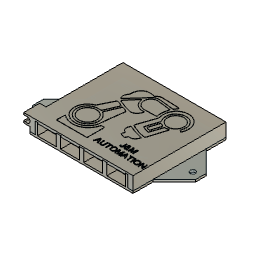
Box for ubs extension cable (Autodesk Fusion 360 design; units mm, degrees)
Autodesk Fusion 360 part; units mm, degrees
(part 1 of 2)
sketch "Sketch1" plane through (0, 0, 0) normal (0, 0, 1) x (1, 0, 0)
  line L0 (0, 0) -> (17, 0)
  line L1 (17, 0) -> (17, 9)
  line L2 (17, 9) -> (0, 9)
  line L3 (0, 9) -> (0, 0)
  line L4 (-0.35, -0.35) -> (17.35, -0.35)
  line L5 (17.35, -0.35) -> (17.35, 9.35)
  line L6 (17.35, 9.35) -> (-0.35, 9.35)
  line L7 (-0.35, 9.35) -> (-0.35, -0.35)
  line L8 (-0.35, 9.35) -> (17.35, 9.35)
  line L9 (17.35, 9.35) -> (17.35, 9.85)
  line L10 (17.35, 9.85) -> (-0.35, 9.85)
  line L11 (-0.35, 9.85) -> (-0.35, 9.35)
  line L12 (-0.35, 9.85) -> (0.65, 9.85)
  line L13 (0.65, 9.85) -> (0.65, 9.35)
  line L14 (0.65, 9.35) -> (-0.35, 9.35)
  line L15 (-0.35, 9.35) -> (-0.35, 9.85)
  line L16 (17.35, 9.85) -> (16.35, 9.85)
  line L17 (16.35, 9.85) -> (16.35, 9.35)
  line L18 (16.35, 9.35) -> (17.35, 9.35)
  line L19 (17.35, 9.35) -> (17.35, 9.85)
  line L20 (17.35, -0.35) -> (19.35, -0.35)
  line L21 (19.35, -0.35) -> (19.35, 9.85)
  line L22 (19.35, 9.85) -> (17.35, 9.85)
  line L23 (17.35, 9.85) -> (17.35, -0.35)
  line L24 (-0.35, -0.35) -> (-2.35, -0.35)
  line L25 (-2.35, -0.35) -> (-2.35, 9.85)
  line L26 (-2.35, 9.85) -> (-0.35, 9.85)
  line L27 (-0.35, 9.85) -> (-0.35, -0.35)
  line L28 (0.65, 9.85) -> (0.65, 9.35)
  line L29 (0.65, 9.35) -> (-0.35, 9.35)
  line L30 (-2.35, -0.35) -> (-2.35, 9.85)
  line L31 (-0.35, 9.85) -> (-0.35, -0.35)
  line L32 (0, 0) -> (17, 0)
  line L33 (17.35, 9.35) -> (17.35, 9.85)
  line L34 (19.35, -0.35) -> (19.35, 9.85)
  line L35 (17.35, -0.35) -> (17.35, 9.35)
  line L36 (17, 0) -> (17, 9)
  line L37 (17, 9) -> (0, 9)
  line L38 (0, 9) -> (0, 0)
  line L39 (-0.35, 9.35) -> (-0.35, -0.35)
  line L40 (17.35, 9.85) -> (-0.35, 9.85)
  line L41 (-0.35, 9.85) -> (-0.35, 9.35)
  line L42 (17.35, 9.85) -> (17.35, -0.35)
  line L43 (-0.35, -0.35) -> (-2.35, -0.35)
  line L44 (17.35, 9.35) -> (-0.35, 9.35)
  line L45 (17.35, 9.85) -> (16.35, 9.85)
  line L46 (-0.35, 9.35) -> (-0.35, 9.85)
  line L47 (17.35, -0.35) -> (19.35, -0.35)
  line L48 (16.35, 9.85) -> (16.35, 9.35)
  line L49 (-0.35, 9.85) -> (0.65, 9.85)
  line L50 (19.35, 9.85) -> (17.35, 9.85)
  line L51 (-2.35, 9.85) -> (-0.35, 9.85)
  line L52 (-0.35, 9.35) -> (17.35, 9.35)
  line L53 (-0.35, -0.35) -> (17.35, -0.35)
  line L54 (17.35, 9.35) -> (17.35, 9.85)
  line L55 (16.35, 9.35) -> (17.35, 9.35)
  line L56 (21.3167, 9.35) -> (21.3167, 9.85)
  line L57 (21.3167, 9.85) -> (22.3167, 9.85)
  line L58 (22.3167, 9.85) -> (22.3167, 9.35)
  line L59 (21.6667, 9) -> (21.6667, 0)
  line L60 (21.6667, 9) -> (21.6667, 0)
  line L61 (21.3167, 9.85) -> (21.3167, 9.35)
  line L62 (19.3167, -0.35) -> (19.3167, 9.85)
  line L63 (21.3167, -0.35) -> (19.3167, -0.35)
  line L64 (19.3167, 9.85) -> (21.3167, 9.85)
  line L65 (22.3167, 9.35) -> (21.3167, 9.35)
  line L66 (21.3167, 9.85) -> (22.3167, 9.85)
  line L67 (19.3167, -0.35) -> (19.3167, 9.85)
  line L68 (21.3167, 9.85) -> (21.3167, -0.35)
  line L69 (21.3167, 9.35) -> (21.3167, -0.35)
  line L70 (21.3167, 9.85) -> (21.3167, 9.35)
  line L71 (21.3167, -0.35) -> (19.3167, -0.35)
  line L72 (38.0167, 9.35) -> (39.0167, 9.35)
  line L73 (39.0167, 9.85) -> (21.3167, 9.85)
  line L74 (41.0167, -0.35) -> (41.0167, 9.85)
  line L75 (19.3167, 9.85) -> (21.3167, 9.85)
  line L76 (39.0167, -0.35) -> (41.0167, -0.35)
  line L77 (21.6667, 0) -> (38.6667, 0)
  line L78 (41.0167, 9.85) -> (39.0167, 9.85)
  line L79 (39.0167, 9.35) -> (21.3167, 9.35)
  line L80 (39.0167, 9.35) -> (39.0167, 9.85)
  line L81 (39.0167, 9.85) -> (39.0167, -0.35)
  line L82 (21.3167, 9.85) -> (21.3167, -0.35)
  line L83 (39.0167, -0.35) -> (39.0167, 9.35)
  line L84 (21.3167, 9.35) -> (21.3167, 9.85)
  line L85 (22.3167, 9.35) -> (21.3167, 9.35)
  line L86 (38.0167, 9.85) -> (38.0167, 9.35)
  line L87 (22.3167, 9.85) -> (22.3167, 9.35)
  line L88 (21.3167, 9.35) -> (21.3167, -0.35)
  line L89 (38.6667, 0) -> (38.6667, 9)
  line L90 (39.0167, -0.35) -> (41.0167, -0.35)
  line L91 (39.0167, 9.35) -> (39.0167, 9.85)
  line L92 (41.0167, -0.35) -> (41.0167, 9.85)
  line L93 (21.6667, 0) -> (38.6667, 0)
  line L94 (39.0167, 9.35) -> (21.3167, 9.35)
  line L95 (38.0167, 9.35) -> (39.0167, 9.35)
  line L96 (38.6667, 9) -> (21.6667, 9)
  line L97 (38.0167, 9.85) -> (38.0167, 9.35)
  line L98 (38.6667, 9) -> (21.6667, 9)
  line L99 (39.0167, 9.35) -> (39.0167, 9.85)
  line L100 (21.3167, 9.35) -> (39.0167, 9.35)
  line L101 (21.3167, -0.35) -> (39.0167, -0.35)
  line L102 (39.0167, -0.35) -> (39.0167, 9.35)
  line L103 (39.0167, 9.85) -> (38.0167, 9.85)
  line L104 (39.0167, 9.85) -> (21.3167, 9.85)
  line L105 (38.6667, 0) -> (38.6667, 9)
  line L106 (41.0167, 9.85) -> (39.0167, 9.85)
  line L107 (39.0167, 9.85) -> (38.0167, 9.85)
  line L108 (39.0167, 9.85) -> (39.0167, -0.35)
  line L109 (39.0167, 9.35) -> (39.0167, 9.85)
  line L110 (21.3167, -0.35) -> (39.0167, -0.35)
  line L111 (21.3167, 9.35) -> (39.0167, 9.35)
  line L112 (42.9833, 9.35) -> (42.9833, 9.85)
  line L113 (42.9833, 9.85) -> (43.9833, 9.85)
  line L114 (43.9833, 9.85) -> (43.9833, 9.35)
  line L115 (43.3333, 9) -> (43.3333, 0)
  line L116 (43.3333, 9) -> (43.3333, 0)
  line L117 (42.9833, 9.85) -> (42.9833, 9.35)
  line L118 (40.9833, -0.35) -> (40.9833, 9.85)
  line L119 (42.9833, -0.35) -> (40.9833, -0.35)
  line L120 (40.9833, 9.85) -> (42.9833, 9.85)
  line L121 (43.9833, 9.35) -> (42.9833, 9.35)
  line L122 (42.9833, 9.85) -> (43.9833, 9.85)
  line L123 (40.9833, -0.35) -> (40.9833, 9.85)
  line L124 (42.9833, 9.85) -> (42.9833, -0.35)
  line L125 (42.9833, 9.35) -> (42.9833, -0.35)
  line L126 (42.9833, 9.85) -> (42.9833, 9.35)
  line L127 (42.9833, -0.35) -> (40.9833, -0.35)
  line L128 (59.6833, 9.35) -> (60.6833, 9.35)
  line L129 (60.6833, 9.85) -> (42.9833, 9.85)
  line L130 (62.6833, -0.35) -> (62.6833, 9.85)
  line L131 (40.9833, 9.85) -> (42.9833, 9.85)
  line L132 (60.6833, -0.35) -> (62.6833, -0.35)
  line L133 (43.3333, 0) -> (60.3333, 0)
  line L134 (62.6833, 9.85) -> (60.6833, 9.85)
  line L135 (60.6833, 9.35) -> (42.9833, 9.35)
  line L136 (60.6833, 9.35) -> (60.6833, 9.85)
  line L137 (60.6833, 9.85) -> (60.6833, -0.35)
  line L138 (42.9833, 9.85) -> (42.9833, -0.35)
  line L139 (60.6833, -0.35) -> (60.6833, 9.35)
  line L140 (42.9833, 9.35) -> (42.9833, 9.85)
  line L141 (43.9833, 9.35) -> (42.9833, 9.35)
  line L142 (59.6833, 9.85) -> (59.6833, 9.35)
  line L143 (43.9833, 9.85) -> (43.9833, 9.35)
  line L144 (42.9833, 9.35) -> (42.9833, -0.35)
  line L145 (60.3333, 0) -> (60.3333, 9)
  line L146 (60.6833, -0.35) -> (62.6833, -0.35)
  line L147 (60.6833, 9.35) -> (60.6833, 9.85)
  line L148 (62.6833, -0.35) -> (62.6833, 9.85)
  line L149 (43.3333, 0) -> (60.3333, 0)
  line L150 (60.6833, 9.35) -> (42.9833, 9.35)
  line L151 (59.6833, 9.35) -> (60.6833, 9.35)
  line L152 (60.3333, 9) -> (43.3333, 9)
  line L153 (59.6833, 9.85) -> (59.6833, 9.35)
  line L154 (60.3333, 9) -> (43.3333, 9)
  line L155 (60.6833, 9.35) -> (60.6833, 9.85)
  line L156 (42.9833, 9.35) -> (60.6833, 9.35)
  line L157 (42.9833, -0.35) -> (60.6833, -0.35)
  line L158 (60.6833, -0.35) -> (60.6833, 9.35)
  line L159 (60.6833, 9.85) -> (59.6833, 9.85)
  line L160 (60.6833, 9.85) -> (42.9833, 9.85)
  line L161 (60.3333, 0) -> (60.3333, 9)
  line L162 (62.6833, 9.85) -> (60.6833, 9.85)
  line L163 (60.6833, 9.85) -> (59.6833, 9.85)
  line L164 (60.6833, 9.85) -> (60.6833, -0.35)
  line L165 (60.6833, 9.35) -> (60.6833, 9.85)
  line L166 (42.9833, -0.35) -> (60.6833, -0.35)
  line L167 (42.9833, 9.35) -> (60.6833, 9.35)
  line L168 (64.65, 9.35) -> (64.65, 9.85)
  line L169 (64.65, 9.85) -> (65.65, 9.85)
  line L170 (65.65, 9.85) -> (65.65, 9.35)
  line L171 (65, 9) -> (65, 0)
  line L172 (65, 9) -> (65, 0)
  line L173 (64.65, 9.85) -> (64.65, 9.35)
  line L174 (62.65, -0.35) -> (62.65, 9.85)
  line L175 (64.65, -0.35) -> (62.65, -0.35)
  line L176 (62.65, 9.85) -> (64.65, 9.85)
  line L177 (65.65, 9.35) -> (64.65, 9.35)
  line L178 (64.65, 9.85) -> (65.65, 9.85)
  line L179 (62.65, -0.35) -> (62.65, 9.85)
  line L180 (64.65, 9.85) -> (64.65, -0.35)
  line L181 (64.65, 9.35) -> (64.65, -0.35)
  line L182 (64.65, 9.85) -> (64.65, 9.35)
  line L183 (64.65, -0.35) -> (62.65, -0.35)
  line L184 (81.35, 9.35) -> (82.35, 9.35)
  line L185 (82.35, 9.85) -> (64.65, 9.85)
  line L186 (84.35, -0.35) -> (84.35, 9.85)
  line L187 (62.65, 9.85) -> (64.65, 9.85)
  line L188 (82.35, -0.35) -> (84.35, -0.35)
  line L189 (65, 0) -> (82, 0)
  line L190 (84.35, 9.85) -> (82.35, 9.85)
  line L191 (82.35, 9.35) -> (64.65, 9.35)
  line L192 (82.35, 9.35) -> (82.35, 9.85)
  line L193 (82.35, 9.85) -> (82.35, -0.35)
  line L194 (64.65, 9.85) -> (64.65, -0.35)
  line L195 (82.35, -0.35) -> (82.35, 9.35)
  line L196 (64.65, 9.35) -> (64.65, 9.85)
  line L197 (65.65, 9.35) -> (64.65, 9.35)
  line L198 (81.35, 9.85) -> (81.35, 9.35)
  line L199 (65.65, 9.85) -> (65.65, 9.35)
  line L200 (64.65, 9.35) -> (64.65, -0.35)
  line L201 (82, 0) -> (82, 9)
  line L202 (82.35, -0.35) -> (84.35, -0.35)
  line L203 (82.35, 9.35) -> (82.35, 9.85)
  line L204 (84.35, -0.35) -> (84.35, 9.85)
  line L205 (65, 0) -> (82, 0)
  line L206 (82.35, 9.35) -> (64.65, 9.35)
  line L207 (81.35, 9.35) -> (82.35, 9.35)
  line L208 (82, 9) -> (65, 9)
  line L209 (81.35, 9.85) -> (81.35, 9.35)
  line L210 (82, 9) -> (65, 9)
  line L211 (82.35, 9.35) -> (82.35, 9.85)
  line L212 (64.65, 9.35) -> (82.35, 9.35)
  line L213 (64.65, -0.35) -> (82.35, -0.35)
  line L214 (82.35, -0.35) -> (82.35, 9.35)
  line L215 (82.35, 9.85) -> (81.35, 9.85)
  line L216 (82.35, 9.85) -> (64.65, 9.85)
  line L217 (82, 0) -> (82, 9)
  line L218 (84.35, 9.85) -> (82.35, 9.85)
  line L219 (82.35, 9.85) -> (81.35, 9.85)
  line L220 (82.35, 9.85) -> (82.35, -0.35)
  line L221 (82.35, 9.35) -> (82.35, 9.85)
  line L222 (64.65, -0.35) -> (82.35, -0.35)
  line L223 (64.65, 9.35) -> (82.35, 9.35)
  line L224 (-2.35, 9.85) -> (84.35, 9.85)
  line L225 (84.35, 9.85) -> (84.35, 79.85)
  line L226 (84.35, 79.85) -> (-2.35, 79.85)
  line L227 (-2.35, 79.85) -> (-2.35, 9.85)
  arc A0 (17.3498, 27.1499) -> (12.4999, 31.9997) centre (12.5001, 27.15) ccw
  arc A1 (4.5, 31.9988) -> (-0.35, 27.1469) centre (4.5, 27.1488) ccw
  arc A2 (4.5, 32.9988) -> (-1.35, 27.1465) centre (4.5, 27.1488) ccw
  arc A3 (18.3501, 27.1499) -> (12.5002, 33) centre (12.5001, 27.15) ccw
  line L228 (4.5, 31.9988) -> (4.5, 32.9988)
  line L229 (-1.35, 27.1465) -> (-0.35, 27.1469)
  arc A4 (40.0168, 27.1499) -> (34.1668, 33) centre (34.1668, 27.15) ccw
  arc A5 (39.0165, 27.1499) -> (34.1666, 31.9997) centre (34.1668, 27.15) ccw
  arc A6 (26.1667, 31.9988) -> (21.3167, 27.1469) centre (26.1667, 27.1488) ccw
  line L230 (26.1667, 31.9988) -> (26.1667, 32.9988)
  arc A7 (26.1667, 32.9988) -> (20.3167, 27.1465) centre (26.1667, 27.1488) ccw
  line L231 (20.3167, 27.1465) -> (21.3167, 27.1469)
  line L232 (60.6832, 27.1499) -> (61.6835, 27.1499)
  arc A8 (61.6835, 27.1499) -> (55.8335, 33) centre (55.8335, 27.15) ccw
  arc A9 (60.6832, 27.1499) -> (55.8332, 31.9997) centre (55.8335, 27.15) ccw
  arc A10 (47.8333, 31.9988) -> (42.9833, 27.1469) centre (47.8333, 27.1488) ccw
  line L233 (47.8333, 31.9988) -> (47.8333, 32.9988)
  arc A11 (47.8333, 32.9988) -> (41.9833, 27.1465) centre (47.8333, 27.1488) ccw
  line L234 (41.9833, 27.1465) -> (42.9833, 27.1469)
  line L235 (82.3498, 27.1499) -> (83.3501, 27.1499)
  arc A12 (83.3501, 27.1499) -> (77.5002, 33) centre (77.5001, 27.15) ccw
  arc A13 (82.3498, 27.1499) -> (77.4999, 31.9997) centre (77.5001, 27.15) ccw
  arc A14 (69.5, 31.9988) -> (64.65, 27.1469) centre (69.5, 27.1488) ccw
  line L236 (69.5, 31.9988) -> (69.5, 32.9988)
  arc A15 (69.5, 32.9988) -> (63.65, 27.1465) centre (69.5, 27.1488) ccw
  line L237 (63.65, 27.1465) -> (64.65, 27.1469)
  line L238 (12.5002, 33) -> (12.4999, 31.9997)
  line L239 (17.3498, 27.1499) -> (18.3501, 27.1499)
  line L240 (39.0165, 27.1499) -> (40.0168, 27.1499)
  line L241 (34.1666, 31.9997) -> (34.1668, 33)
  line L242 (55.8332, 31.9997) -> (55.8335, 33)
  line L243 (77.4999, 31.9997) -> (77.5002, 33)
  line L244 (-2.35, 79.85) -> (84.35, 79.85)
  line L245 (84.35, 79.85) -> (84.35, 81.85)
  line L246 (84.35, 81.85) -> (-2.35, 81.85)
  line L247 (-2.35, 81.85) -> (-2.35, 79.85)
  line L248 (-2.35, 9.85) -> (-0.35, 9.85)
  line L249 (-0.35, 9.85) -> (-0.35, 9.6)
  line L250 (-0.35, 9.6) -> (-2.35, 9.6)
  line L251 (-2.35, 9.6) -> (-2.35, 9.85)
  line L252 (17.35, 9.85) -> (21.3167, 9.85)
  line L253 (21.3167, 9.85) -> (21.3167, 9.5)
  line L254 (21.3167, 9.5) -> (17.35, 9.5)
  line L255 (17.35, 9.5) -> (17.35, 9.85)
  line L256 (39.0167, 9.85) -> (42.9833, 9.85)
  line L257 (42.9833, 9.85) -> (42.9833, 9.5)
  line L258 (42.9833, 9.5) -> (39.0167, 9.5)
  line L259 (39.0167, 9.5) -> (39.0167, 9.85)
  line L260 (60.6833, 9.85) -> (64.65, 9.85)
  line L261 (64.65, 9.85) -> (64.65, 9.5)
  line L262 (64.65, 9.5) -> (60.6833, 9.5)
  line L263 (60.6833, 9.5) -> (60.6833, 9.85)
  line L264 (82.35, 9.85) -> (84.35, 9.85)
  line L265 (84.35, 9.85) -> (84.35, 9.5)
  line L266 (84.35, 9.5) -> (82.35, 9.5)
  line L267 (82.35, 9.5) -> (82.35, 9.85)
  line L268 (84.35, 79.85) -> (-2.35, 79.85)
  line L269 (-2.35, 79.85) -> (-2.35, 80.2)
  line L270 (-2.35, 80.2) -> (84.35, 80.2)
  line L271 (84.35, 80.2) -> (84.35, 79.85)
  line L272 (84.35, -0.35) -> (89.35, -0.35)
  line L273 (89.35, -0.35) -> (89.35, 81.85)
  line L274 (89.35, 81.85) -> (84.35, 81.85)
  line L275 (84.35, 81.85) -> (84.35, -0.35)
  line L276 (-2.35, -0.35) -> (-7.35, -0.35)
  line L277 (-7.35, -0.35) -> (-7.35, 81.85)
  line L278 (-7.35, 81.85) -> (-2.35, 81.85)
  line L279 (-2.35, 81.85) -> (-2.35, -0.35)
  line L280 (-7.35, 81.85) -> (89.35, 81.85)
  line L281 (89.35, 81.85) -> (89.35, 86.85)
  line L282 (89.35, 86.85) -> (-7.35, 86.85)
  line L283 (-7.35, 86.85) -> (-7.35, 81.85)
  line L284 (-7.35, -0.35) -> (89.35, -0.35)
  line L285 (89.35, 48.25) -> (109.35, 48.25)
  line L286 (109.35, 48.25) -> (109.35, 38.25)
  line L287 (109.35, 38.25) -> (89.35, 38.25)
  line L288 (89.35, 38.25) -> (89.35, 48.25)
  line L289 (89.35, 18.25) -> (109.35, 38.25)
  line L290 (109.35, 48.25) -> (89.35, 68.25)
  circle A16 centre (101.85, 43.25) radius 2.5
  line L291 (-7.35, 22.0462) -> (-27.35, 22.0462)
  line L292 (-27.35, 22.0462) -> (-27.35, 32.0462)
  line L293 (-27.35, 32.0462) -> (-7.35, 32.0462)
  line L294 (-7.35, 32.0462) -> (-7.35, 22.0462)
  line L295 (-27.35, 22.0462) -> (-7.35, 2.0462)
  line L296 (-27.35, 32.0462) -> (-7.35, 52.0462)
  circle A17 centre (-19.85, 43.25) radius 2.5
  point P0 (21.6667, 0)
  point P1 (21.6667, 0)
  point P2 (43.3333, 0)
  point P3 (43.3333, 0)
  point P4 (65, 0)
  point P5 (65, 0)
  dimension "d1" = 17
  dimension "d2" = 9
  dimension "d3" = 0.35
  dimension "d4" = 0.5
  dimension "d5" = 1
  dimension "d6" = 1
  dimension "d7" = 2
  dimension "d8" = 2
  dimension "d9" = 0.35
  dimension "d10" = 17
  dimension "d11" = 9
  dimension "d12" = 0.5
  dimension "d13" = 1
  dimension "d14" = 1
  dimension "d15" = 2
  dimension "d16" = 2
  dimension "d19" = 65
  dimension "d20" = 0
  dimension "d27" = 70
  dimension "d41" = 5.85
  dimension "d42" = 5.85
  dimension "d52" = 2
  dimension "d67" = 0.25
  dimension "d68" = 0.35
  dimension "d69" = 0.35
  dimension "d70" = 0.35
  dimension "d71" = 0.35
  dimension "d72" = 0.35
  dimension "d73" = 5
  dimension "d74" = 5
  dimension "d75" = 5
  dimension "d93" = 20
  dimension "d94" = 10
  dimension "d95" = 38.6
  dimension "d96" = 45
  dimension "d97" = 45
  dimension "d98" = 5
  dimension "d99" = 7.5
  dimension "d100" = 20
  dimension "d101" = 10
  dimension "d102" = 45
  dimension "d103" = 45
  dimension "d104" = 5
  dimension "d105" = 7.5
  constraint horizontal L0
  constraint vertical L1
  constraint horizontal L2
  constraint vertical L3
  constraint coincident L0.start L3.end
  constraint horizontal L8
  constraint vertical L9
  constraint horizontal L10
  constraint vertical L11
  constraint horizontal L12
  constraint vertical L13
  constraint horizontal L14
  constraint vertical L15
  constraint horizontal L16
  constraint vertical L17
  constraint horizontal L18
  constraint vertical L19
  constraint horizontal L20
  constraint vertical L21
  constraint horizontal L22
  constraint vertical L23
  constraint horizontal L24
  constraint vertical L25
  constraint horizontal L26
  constraint vertical L27
  constraint horizontal L32
  constraint vertical L36
  constraint horizontal L37
  constraint vertical L38
  constraint horizontal L52
  constraint vertical L54
  constraint horizontal L40
  constraint vertical L41
  constraint horizontal L49
  constraint vertical L28
  constraint horizontal L29
  constraint vertical L46
  constraint horizontal L45
  constraint vertical L48
  constraint horizontal L55
  constraint vertical L33
  constraint horizontal L47
  constraint vertical L34
  constraint horizontal L50
  constraint vertical L42
  constraint horizontal L43
  constraint vertical L30
  constraint horizontal L51
  constraint vertical L31
  constraint horizontal L224
  constraint vertical L225
  constraint horizontal L226
  constraint vertical L227
  constraint coincident A1.centre A2.centre
  constraint coincident A0.centre A3.centre
  constraint horizontal L244
  constraint vertical L245
  constraint horizontal L246
  constraint vertical L247
  constraint horizontal L248
  constraint vertical L249
  constraint horizontal L250
  constraint vertical L251
  constraint horizontal L252
  constraint vertical L253
  constraint horizontal L254
  constraint vertical L255
  constraint horizontal L256
  constraint vertical L257
  constraint horizontal L258
  constraint vertical L259
  constraint horizontal L260
  constraint vertical L261
  constraint horizontal L262
  constraint vertical L263
  constraint horizontal L264
  constraint vertical L265
  constraint horizontal L266
  constraint vertical L267
  constraint coincident L186 L265.end
  constraint horizontal L268
  constraint vertical L269
  constraint horizontal L270
  constraint vertical L271
  constraint horizontal L272
  constraint vertical L273
  constraint horizontal L274
  constraint vertical L275
  constraint horizontal L276
  constraint vertical L277
  constraint horizontal L278
  constraint vertical L279
  constraint horizontal L280
  constraint vertical L281
  constraint horizontal L282
  constraint vertical L283
  constraint horizontal L284
  constraint horizontal L285
  constraint vertical L286
  constraint horizontal L287
  constraint vertical L288
  constraint coincident L273 L285.start
  constraint coincident L273 L289.start
  constraint coincident L273 L290.end
  constraint horizontal L291
  constraint vertical L292
  constraint horizontal L293
  constraint vertical L294
  constraint coincident L277 L291.start
  constraint coincident L277 L295.end
  constraint coincident L277 L296.end
  measures "d1" distance of L0.start L0.end
  measures "d2" distance of L0.start L2.end
  measures "d4" distance of L6.end L10.end
  measures "d5" distance of L10.end L12.end
  measures "d6" distance of L9.end L16.end
  measures "d7" distance of L4.end L20.end
  measures "d8" distance of L4.start L24.end
  measures "d10" distance of L0.start L0.end
  measures "d11" distance of L0.start L2.end
  measures "d12" distance of L10.end L6.end
  measures "d13" distance of L10.end L12.end
  measures "d14" distance of L9.end L16.end
  measures "d15" distance of L4.end L20.end
  measures "d16" distance of L24.end L4.start
  measures "d27" distance of L25.end L226.end
  measures "d41" radius of A2
  measures "d42" radius of A3
  measures "d52" distance of L226.end L246.end
  measures "d67" distance of L25.end L250.end
  measures "d68" distance of L9.end L254.end
  measures "d69" distance of L73.start L258.end
  measures "d70" distance of L129.start L262.end
  measures "d71" distance of L185.start L266.end
  measures "d72" distance of L225.end L270.end
  measures "d73" distance of L186.start L272.end
  measures "d74" distance of L24.end L276.end
  measures "d75" distance of L277.end L282.end
  measures "d93" distance of L285.start L285.end
  measures "d94" distance of L285.start L287.end
  measures "d95" distance of L284 L287
  measures "d96" angle of L273 L289
  measures "d97" angle of L273 L290
  measures "d98" diameter of A16
  measures "d99" distance of L286 A16.centre
  measures "d100" distance of L291.start L291.end
  measures "d101" distance of L291.start L293.end
  measures "d102" angle of L277 L296
  measures "d103" angle of L277 L295
  measures "d104" diameter of A17
  measures "d105" distance of L292 A17.centre
extrude "Extrude1" add sketch "Sketch1" along normal blind 2 contours L0 L1 L2 L3 L32 L36 L37 L38 | L4 L5 L6 L7 L8 L14 L18 L23 L27 L29 L31 L35 L39 L42 L44 L52 L53 L55 L284 | L25 L30 L227 L247 L251 L269 L276 L277 L278 L279 L280 L284 L294 | L10 L12 L16 L22 L26 L40 L45 L49 L50 L51 L57 L64 L66 L73 L75 L78 L103 L104 L106 L107 L113 L120 L122 L129 L131 L134 L159 L160 L162 L163 L169 L176 L178 L185 L187 L190 L215 L216 L218 L219 L224 L225 L226 L227 L244 L248 L252 L256 L260 L264 L268 L275 L279 | L277 L291 L295 | L65 L68 L69 L72 L79 L81 L82 L83 L85 L88 L94 L95 L100 L101 L102 L108 L110 L111 L284 | L277 L291 L292 L293 L294 | L186 L204 L225 L245 L265 L271 L272 L273 L274 L275 L280 L284 L288 | L277 L293 L296 | L246 L274 L278 L280 L281 L282 L283 | L121 L124 L125 L128 L135 L137 L138 L139 L141 L144 L150 L151 L156 L157 L158 L164 L166 L167 L284 | L177 L180 L181 L184 L191 L193 L194 L195 L197 L200 L206 L207 L212 L213 L214 L220 L222 L223 L284 | L273 L285 L290 | L273 L287 L289 | L273 L285 L286 L287 L288 | L59 L60 L77 L89 L93 L96 L98 L105 | L115 L116 L133 L145 L149 L152 L154 L161 | L171 L172 L189 L201 L205 L208 L210 L217 makes body 1 at (38.9998, 64.2135, 0) makes body 2 at (27.2167, 6.1167, 0) makes body 3 at (5.55, 2.8833, 0) makes body 4 at (48.8833, 2.8833, 0) makes body 5 at (70.55, 2.8833, 0)
extrude "Extrude2" add sketch "Sketch1" along normal blind 13 contours L7 L11 L15 L24 L25 L27 L30 L31 L39 L41 L43 L46 L250 L279 L284 | L5 L9 L19 L20 L23 L33 L35 L42 L47 L54 L62 L67 L254 L284 | L20 L21 L34 L47 L62 L63 L67 L71 L254 L284 | L21 L34 L56 L61 L63 L68 L69 L70 L71 L82 L84 L88 L254 L284 | L21 L22 L34 L50 L62 L64 L67 L75 L224 L252 L254 | L76 L80 L81 L83 L90 L91 L99 L102 L108 L109 L118 L123 L258 L284 | L245 L246 L247 L270 L275 L279 L280 | L74 L76 L90 L92 L118 L119 L123 L127 L258 L284 | L74 L92 L112 L117 L119 L124 L125 L126 L127 L138 L140 L144 L258 L284 | L74 L78 L92 L106 L118 L120 L123 L131 L224 L256 L258 | L186 L188 L192 L193 L195 L202 L203 L204 L211 L214 L220 L221 L266 L275 L284 | L132 L136 L137 L139 L146 L147 L155 L158 L164 L165 L174 L179 L262 L284 | L130 L132 L146 L148 L174 L175 L179 L183 L262 L284 | L130 L148 L168 L173 L175 L180 L181 L182 L183 L194 L196 L200 L262 L284 | L130 L134 L148 L162 L174 L176 L179 L187 L224 L260 L262 bodies 1 2 4 5 3
extrude "Extrude3" add sketch "Sketch1" along normal blind 3 contours L6 L8 L10 L13 L17 L28 L40 L44 L48 L52 L224 | L58 L73 L79 L86 L87 L94 L97 L100 L104 L111 L224 | L170 L185 L191 L198 L199 L206 L209 L212 L216 L223 L224 | L114 L129 L135 L142 L143 L150 L153 L156 L160 L167 L224 bodies 1
extrude "Extrude4" add sketch "Sketch1" along normal blind 8 contours A0 A3 L238 L239 | A1 A2 L228 L229 | A4 A5 L240 L241 | A6 L230 A7 L231 | L232 A8 A9 L242 | A10 L233 A11 L234 | L235 A12 A13 L243 | A14 L236 A15 L237 bodies 1
extrude "Extrude5" add sketch "Sketch1" along normal blind 12 contours L6 L8 L10 L11 L12 L13 L14 L15 L27 L28 L29 L31 L40 L41 L44 L46 L49 L52 L224 L249 | L6 L8 L9 L10 L16 L17 L18 L19 L23 L33 L40 L42 L44 L45 L48 L52 L54 L55 L224 L255 | L11 L15 L25 L26 L27 L30 L31 L41 L46 L51 L224 L248 L249 L250 L251 L279 | L9 L19 L22 L23 L33 L42 L50 L54 L62 L67 L224 L252 L254 L255 | L21 L34 L56 L61 L64 L68 L70 L75 L82 L84 L224 L252 L253 L254 | L226 L244 L245 L247 L268 L269 L270 L271 L275 L279 | L56 L57 L58 L61 L65 L66 L68 L70 L73 L79 L82 L84 L85 L87 L94 L100 L104 L111 L224 L253 | L72 L73 L79 L80 L81 L86 L91 L94 L95 L97 L99 L100 L103 L104 L107 L108 L109 L111 L224 L259 | L186 L190 L192 L193 L203 L204 L211 L218 L220 L221 L224 L264 L265 L266 L267 L275 | L78 L80 L81 L91 L99 L106 L108 L109 L118 L123 L224 L256 L258 L259 | L184 L185 L191 L192 L193 L198 L203 L206 L207 L209 L211 L212 L215 L216 L219 L220 L221 L223 L224 L267 | L74 L92 L112 L117 L120 L124 L126 L131 L138 L140 L224 L256 L257 L258 | L112 L113 L114 L117 L121 L122 L124 L126 L129 L135 L138 L140 L141 L143 L150 L156 L160 L167 L224 L257 | L168 L169 L170 L173 L177 L178 L180 L182 L185 L191 L194 L196 L197 L199 L206 L212 L216 L223 L224 L261 | L128 L129 L135 L136 L137 L142 L147 L150 L151 L153 L155 L156 L159 L160 L163 L164 L165 L167 L224 L263 | L130 L148 L168 L173 L176 L180 L182 L187 L194 L196 L224 L260 L261 L262 | L134 L136 L137 L147 L155 L162 L164 L165 L174 L179 L224 L260 L262 L263 bodies 1
sketch "Sketch2" plane through (0, 0, 13) normal (0, 0, 1) x (-1, 0, 0)
  line L0 (2.35, -81.85) -> (2.35, -80.2)
  line L1 (-84.35, -80.2) -> (-84.35, -81.85)
  line L2 (-84.35, -81.85) -> (2.35, -81.85)
  line L3 (2.35, -81.85) -> (-84.35, -81.85)
  line L4 (-84.35, -81.85) -> (-84.35, 0.35)
  line L5 (-84.35, 0.35) -> (2.35, 0.35)
  line L6 (2.35, 0.35) -> (2.35, -81.85)
  line L7 (2.35, -80.2) -> (-84.35, -80.2)
  constraint horizontal L3
  constraint vertical L4
  constraint horizontal L5
  constraint vertical L6
  constraint coincident L0.start L2.end
extrude "Extrude6" add sketch "Sketch2" along normal blind 2.5 separate body makes body 6
sketch "Sketch3" plane through (0, 0, 13) normal (0, 0, -1) x (1, 0, 0)
  line L0 (84.35, 0.35) -> (-2.35, 0.35)
  line L1 (-2.35, 0.35) -> (-2.35, -81.85)
  line L2 (84.35, -81.85) -> (84.35, 0.35)
  line L3 (-2.35, 0.35) -> (0, 0.35)
  line L4 (0, 0.35) -> (0, -9.85)
  line L5 (0, -9.85) -> (-2.35, -9.85)
  line L6 (-2.35, -9.85) -> (-2.35, 0.35)
  line L7 (0, 0.35) -> (17, 0.35)
  line L8 (17, 0.35) -> (21.6675, 0.35)
  line L9 (21.6675, 0.35) -> (21.6675, -9.85)
  line L10 (21.6675, -9.85) -> (17, -9.85)
  line L11 (17, -9.85) -> (17, 0.35)
  line L12 (38.6675, 0.35) -> (43.335, 0.35)
  line L13 (38.6675, -9.85) -> (38.6675, 0.35)
  line L14 (43.335, 0.35) -> (43.335, -9.85)
  line L15 (43.335, -9.85) -> (38.6675, -9.85)
  line L16 (60.335, 0.35) -> (65.0025, 0.35)
  line L17 (60.335, -9.85) -> (60.335, 0.35)
  line L18 (65.0025, 0.35) -> (65.0025, -9.85)
  line L19 (65.0025, -9.85) -> (60.335, -9.85)
  line L20 (84.35, 0.35) -> (82, 0.35)
  line L21 (82, 0.35) -> (82, -9.85)
  line L22 (82, -9.85) -> (84.35, -9.85)
  line L23 (84.35, -9.85) -> (84.35, 0.35)
  line L24 (-2.35, -81.85) -> (84.35, -81.85)
  line L25 (-2.35, -81.85) -> (-2.35, -79.85)
  line L26 (-2.35, -79.85) -> (84.35, -79.85)
  line L27 (84.35, -81.85) -> (84.35, -79.85)
  line L28 (-2.35, -81.85) -> (-7.35, -81.85)
  line L29 (-7.35, -81.85) -> (-7.35, 0.35)
  line L30 (-7.35, 0.35) -> (-2.35, 0.35)
  line L31 (-2.35, 0.35) -> (-2.35, -81.85)
  line L32 (84.35, 0.35) -> (89.35, 0.35)
  line L33 (89.35, 0.35) -> (89.35, -81.85)
  line L34 (89.35, -81.85) -> (84.35, -81.85)
  line L35 (84.35, -81.85) -> (84.35, 0.35)
  line L36 (-7.35, 0.35) -> (89.35, 0.35)
  line L37 (-7.35, -81.85) -> (89.35, -81.85)
  line L38 (89.35, -81.85) -> (89.35, -86.85)
  line L39 (89.35, -86.85) -> (-7.35, -86.85)
  line L40 (-7.35, -86.85) -> (-7.35, -81.85)
  line L41 (-2.35, 0.35) -> (-2.7, 0.35)
  line L42 (-2.7, 0.35) -> (-2.7, -81.85)
  line L43 (-2.7, -81.85) -> (-2.35, -81.85)
  line L44 (-2.35, -81.85) -> (-2.35, 0.35)
  line L45 (84.35, 0.35) -> (84.7, 0.35)
  line L46 (84.7, 0.35) -> (84.7, -81.85)
  line L47 (84.7, -81.85) -> (84.35, -81.85)
  line L48 (84.35, -81.85) -> (84.35, 0.35)
  line L49 (-2.7, 0.35) -> (84.7, 0.35)
  line L50 (-2.7, -81.85) -> (84.7, -81.85)
  line L51 (84.7, -81.85) -> (84.7, -82.2)
  line L52 (84.7, -82.2) -> (-2.7, -82.2)
  line L53 (-2.7, -82.2) -> (-2.7, -81.85)
  dimension "d55" = 2.35
  dimension "d56" = 10.2
  dimension "d57" = 10.2
  dimension "d60" = 43.335
  dimension "d61" = 0
  dimension "d62" = 10.2
  dimension "d66" = 2
  dimension "d77" = 5
  dimension "d78" = 5
  dimension "d80" = 5
  dimension "d85" = 0.35
  dimension "d86" = 0.35
  dimension "d88" = 0.35
  constraint horizontal L3
  constraint vertical L4
  constraint horizontal L5
  constraint vertical L6
  constraint coincident L0.end L1.start
  constraint coincident L0 L7.end
  constraint horizontal L8
  constraint vertical L9
  constraint horizontal L10
  constraint vertical L11
  constraint horizontal L20
  constraint vertical L21
  constraint horizontal L22
  constraint vertical L23
  constraint coincident L0.start L2.end
  constraint coincident L1.end L24.start
  constraint perpendicular L24 L25
  constraint coincident L2 L26.end
  constraint perpendicular L2 L26
  constraint coincident L2.start L24.end
  constraint horizontal L28
  constraint vertical L29
  constraint horizontal L30
  constraint vertical L31
  constraint horizontal L32
  constraint vertical L33
  constraint horizontal L34
  constraint vertical L35
  constraint horizontal L36
  constraint horizontal L37
  constraint vertical L38
  constraint horizontal L39
  constraint vertical L40
  constraint horizontal L41
  constraint vertical L42
  constraint horizontal L43
  constraint vertical L44
  constraint horizontal L45
  constraint vertical L46
  constraint horizontal L47
  constraint vertical L48
  constraint horizontal L49
  constraint horizontal L50
  constraint vertical L51
  constraint horizontal L52
  constraint vertical L53
  measures "d55" distance of L0.end L3.end
  measures "d56" distance of L0.end L5.end
  measures "d57" distance of L7.end L10.end
  measures "d62" distance of L0.start L22.end
  measures "d66" distance of L1.end L25.end
  measures "d77" distance of L1.end L28.end
  measures "d78" distance of L0.start L32.end
  measures "d80" distance of L28.end L39.end
  measures "d85" distance of L0.end L41.end
  measures "d86" distance of L0.start L45.end
  measures "d88" distance of L42.end L52.end
extrude "Extrude7" cut sketch "Sketch3" against normal blind 1 contours L0 L2 L20 L21 L22 L23 L35 L36 L48 L49 | L0 L16 L17 L18 L19 L36 L49 | L1 L2 L24 L25 L26 L27 L31 L35 L37 L44 L48 L50 | L0 L12 L13 L14 L15 L36 L49 | L0 L1 L3 L4 L5 L6 L31 L36 L44 L49 | L0 L8 L9 L10 L11 L36 L49 bodies 6
copy_body "Body->Comp1" bodies 1 removing the originals makes body 7 in component "boksi"
copy_body "Body->Comp2" bodies 6 removing the originals makes body 8 in component "kansi"
extrude "Extrude1'" add sketch "Sketch3" along normal blind 11 and the other way blind 1.5 contours L2 L23 L27 L32 L34 L35 L36 L37 L45 L46 L47 L48 L49 L50 | L32 L33 L34 L36 L37 L46 | L24 L28 L34 L37 L43 L47 L50 L51 L52 L53 | L28 L34 L37 L38 L39 L40 L51 L52 L53 | L1 L6 L25 L28 L30 L31 L36 L37 L41 L42 L43 L44 L49 L50 | L28 L29 L30 L36 L37 L42 sketch seen with x (1, 0, 0) y (0, 1, 0) z (0, 0, 1) at (0, 0, 1) bodies 8 in component "kansi"
sketch "Sketch4" plane through (0, 0, 0) normal (0, 0, -1) x (1, 0, 0)
  line L0 (89.35, 0.35) -> (-7.35, 0.35)
  line L1 (-7.35, 0.35) -> (-7.35, -2.0462)
  line L2 (-7.35, -2.0462) -> (-27.35, -22.0462)
  line L3 (-27.35, -22.0462) -> (-27.35, -32.0462)
  line L4 (-27.35, -32.0462) -> (-7.35, -52.0462)
  line L5 (-7.35, -52.0462) -> (-7.35, -86.85)
  line L6 (-7.35, -86.85) -> (89.35, -86.85)
  line L7 (89.35, -86.85) -> (89.35, -68.25)
  line L8 (89.35, -68.25) -> (109.35, -48.25)
  line L9 (109.35, -48.25) -> (109.35, -38.25)
  line L10 (109.35, -38.25) -> (89.35, -18.25)
  line L11 (89.35, -18.25) -> (89.35, 0.35)
  circle A0 centre (101.85, -43.25) radius 2.5
  circle A1 centre (86.85, -29.65) radius 1.5
  circle A2 centre (-4.85, -29.65) radius 1.5
  circle A3 centre (-4.85, -56.85) radius 1.5
  circle A4 centre (86.85, -56.85) radius 1.5
  circle A5 centre (86.85, -56.85) radius 2.2
  circle A6 centre (86.85, -29.65) radius 2.2
  circle A7 centre (-4.85, -29.65) radius 2.2
  circle A8 centre (-4.85, -56.85) radius 2.2
  dimension "d106" = 3
  dimension "d107" = 2.5
  dimension "d108" = 30
  dimension "d109" = 3
  dimension "d110" = 2.5
  dimension "d111" = 30
  dimension "d112" = 3
  dimension "d113" = 30
  dimension "d114" = 2.5
  dimension "d115" = 3
  dimension "d116" = 30
  dimension "d117" = 2.5
  dimension "d118" = 4.4
  dimension "d119" = 4.4
  dimension "d120" = 4.4
  dimension "d121" = 4.4
  constraint concentric A4 A5
  constraint concentric A1 A6
  constraint concentric A2 A7
  constraint concentric A3 A8
  measures "d106" diameter of A1
  measures "d107" distance of L11 A1.centre
  measures "d108" distance of L0 A1.centre
  measures "d109" diameter of A2
  measures "d110" distance of L1 A2.centre
  measures "d111" distance of L0 A2.centre
  measures "d112" diameter of A3
  measures "d113" distance of L6 A3.centre
  measures "d114" distance of L5 A3.centre
  measures "d115" diameter of A4
  measures "d116" distance of L6 A4.centre
  measures "d117" distance of L7 A4.centre
  measures "d118" diameter of A5
  measures "d119" diameter of A6
  measures "d120" diameter of A7
  measures "d121" diameter of A8
extrude "Extrude1''" cut sketch "Sketch4" against normal blind 8 contours A1 | A2 | A3 | A4 bodies 7 in component "boksi"
extrude "Extrude3'" cut sketch "Sketch4" against normal blind 8 contours A1 | A2 | A3 | A4 sketch seen with x (1, 0, 0) y (0, 1, 0) z (0, 0, 1) at (0, 0, 1) bodies 8 in component "kansi"
extrude "Extrude2'" cut sketch "Sketch4" against normal blind 1 contours A5 | A6 | A7 | A8 bodies 7 in component "boksi"